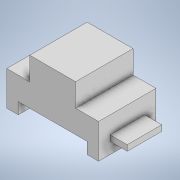
# Autodesk Inventor part: 4.2 Part A
Saved by Autodesk Inventor 2020 (Build 240168000, 168)
## iProperties
Created: 2020-01-07
Part Number: 4.2 Part A
Material: Generic
Document SubType Name: Modeling
Designer: cks4a449
Density: 1 g/cm^3
Appearance: Default
Author: cks4a449
Autodesk Inventor part; units mm, degrees
ref_plane "YZ Plane" through (0, 0, 0) normal (1, 0, 0) x (0, 1, 0)
ref_plane "XZ Plane" through (0, 0, 0) normal (0, 1, 0) x (-1, 0, 0)
ref_plane "XY Plane" through (0, 0, 0) normal (0, 0, 1) x (1, 0, 0)
sketch "Sketch1" plane through (0, 0, 0) normal (0, 1, 0) x (-1, 0, 0)
  line L0 (-101.6, 0) -> (-101.6, -38.1)
  line L1 (-76.2, -63.5) -> (-25.4, -63.5)
  line L2 (-88.9, 0) -> (-88.9, -12.7)
  line L3 (-88.9, -12.7) -> (-12.7, -12.7)
  line L4 (-12.7, -12.7) -> (-12.7, 0)
  line L5 (-25.4, -63.5) -> (-25.4, -38.1)
  line L6 (-25.4, -38.1) -> (0, -38.1)
  line L7 (-76.2, -63.5) -> (-76.2, -38.1)
  line L8 (-76.2, -38.1) -> (-101.6, -38.1)
  line L9 (-88.9, 0) -> (-101.6, 0)
  line L10 (0, -38.1) -> (0, 0)
  line L11 (0, 0) -> (-12.7, 0)
  dimension "d2" = 76.2
  dimension "d3" = 12.7
  dimension "d4" = 25.4
  dimension "d5" = 25.4
  dimension "d6" = 25.4
  dimension "d7" = 25.4
  dimension "d8" = 38.1
  constraints: 24 end point, 2 parallel, 2 perpendicular, 1 horizontal, 1 vertical
  measures "d2" distance of L3.end L2.end
  measures "d3" distance of L2.end L2.start
  measures "d4" distance of L6.end L5.end
  measures "d5" distance of L1.end L5.end
  measures "d6" distance of L0.end L7.end
  measures "d7" distance of L1.start L7.end
  measures "d8" distance of L6.end L10.end
extrude "Extrusion1" add sketch "Sketch1" along normal blind 63.5
sketch "Sketch2" plane through (101.6, 0, 0) normal (1, 0, 0) x (0, 0, -1)
  line L0 (63.5, 63.5) -> (38.1, 63.5) projected
  line L1 (19.05, 50.8) -> (12.7, 50.8)
  line L2 (12.7, 50.8) -> (12.7, 12.7)
  line L3 (12.7, 12.7) -> (19.05, 12.7)
  line L4 (19.05, 12.7) -> (19.05, 50.8)
  point P0 (0, 63.5)
  dimension "d14" = 6.35
  dimension "d15" = 38.1
  constraints: 8 end point, 2 parallel, 1 horizontal, 1 perpendicular
  measures "d14" distance of L3.end L2.end
  measures "d15" distance of L2.end L1.end
extrude "Extrusion2" add sketch "Sketch2" along normal blind 19.05
body "Solid1"
